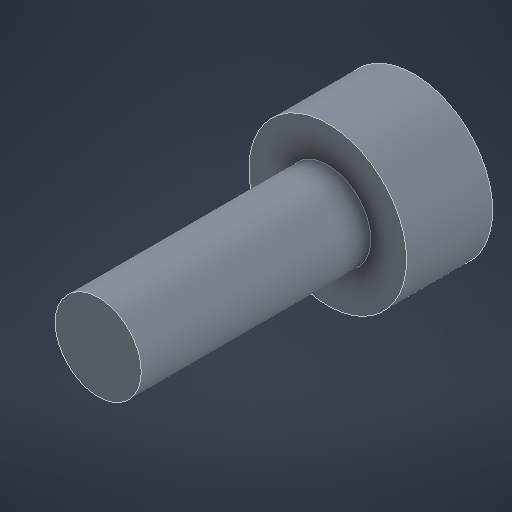
# Autodesk Inventor part: Rod_M3x8_Simplified
Saved by Autodesk Inventor 2027.1 (Build 311270010, 270A)
## iProperties
Created: 2026-09-21
Part Number: Rod_M3x8_Simplified
Material: Generic
Document SubType Name: Modeling
Designer: 박정현
Density: 1 g/cm^3
Appearance: Simplified fastener
Author: 박정현
Comments: Illustrative M3 x 8 socket-head fastener envelope, 5.5 mm head diameter and 3 mm head height. Threads omitted; engaged region shown at bore diameter to avoid false interference. Verify fastener specification and engagement before fabrication.
Autodesk Inventor part; units mm, degrees
ref_plane "Work Plane1" through (0, 0, -3) normal (0, 0, 1) x (1, 0, 0)
sketch "Sketch1" plane through (0, 0, -3) normal (0, 0, 1) x (1, 0, 0)
  circle A0 centre (0, 0) radius 2.75
  constraints: 1 centre point
extrude "M3_Head_Envelope" add sketch "Sketch1" along normal blind 3
sketch "Sketch2" plane through (0, 0, 0) normal (0, 0, 1) x (1, 0, 0)
  circle A0 centre (0, 0) radius 1.5
  constraints: 1 centre point
extrude "M3_Clearance_Grip" add sketch "Sketch2" along normal blind 4
ref_plane "Work Plane2" through (0, 0, 4) normal (0, 0, 1) x (1, 0, 0)
sketch "Sketch3" plane through (0, 0, 4) normal (0, 0, 1) x (1, 0, 0)
  circle A0 centre (0, 0) radius 1.5
  constraints: 1 centre point
extrude "Thread_Core_No_Helix" add sketch "Sketch3" along normal blind 4
ref_plane "Work Plane3" through (0, 0, -3) normal (0, 0, 1) x (1, 0, 0)
sketch "Sketch4" plane through (0, 0, -3) normal (0, 0, 1) x (1, 0, 0)
  circle A0 centre (0, 0) radius 1.25
  constraints: 1 centre point
extrude "Extrusion4" cut sketch "Sketch4" along normal blind 1.5
body "Solid1"
